Autodesk Fusion 360 part; units mm, degrees
(part 4 of 4)
  constraint vertical L97
  constraint horizontal L47
  constraint vertical L93
  constraint coincident L93.end L232
  constraint coincident L93.end L237
  constraint horizontal L222
  constraint vertical L60
  constraint horizontal L64
  constraint vertical L236
  constraint coincident L222.start L207
  constraint coincident L222.start L231
  constraint horizontal L71
  constraint vertical L234
  constraint horizontal L88
  constraint vertical L148
  constraint coincident L71.start L207
  constraint coincident L71.start L213
  constraint horizontal L81
  constraint vertical L221
  constraint horizontal L149
  constraint vertical L77
  constraint horizontal L65
  constraint vertical L68
  constraint horizontal L66
  constraint vertical L59
  constraint horizontal L104
  constraint vertical L118
  constraint horizontal L18
  constraint vertical L109
  constraint coincident L104.start L207
  constraint coincident L104.start L107
  constraint horizontal L113
  constraint vertical L55
  constraint horizontal L111
  constraint vertical L116
  constraint horizontal L58
  constraint vertical L105
  constraint horizontal L115
  constraint vertical L19
  constraint horizontal L37
  constraint vertical L45
  constraint horizontal L227
  constraint vertical L53
  constraint horizontal L99
  constraint vertical L46
  constraint horizontal L41
  constraint vertical L49
  constraint horizontal L75
  constraint vertical L67
  constraint horizontal L244
  constraint vertical L70
  constraint horizontal L73
  constraint vertical L72
  constraint horizontal L220
  constraint vertical L224
  constraint coincident L73.start L219.start
  constraint coincident P0 L239.start
  constraint perpendicular L223 L239
  constraint coincident A35.centre L240
  constraint coincident A35 L240.end
  constraint coincident A35 L241.start
  constraint collinear L240 L241
  constraint coincident A36.centre L241
  constraint coincident A36 L241.end
  constraint coincident A36 L242.start
  constraint collinear L241 L242
  constraint coincident A37.centre L242
  constraint coincident A37 L242.end
  constraint coincident A37 L243.start
  constraint collinear L242 L243
  constraint coincident A38.centre L243
  constraint coincident A38 L243.end
  constraint coincident A38 L246.start
  constraint collinear L243 L246
  constraint coincident A39.centre L246
  constraint coincident A40.centre L246
  constraint coincident A40 L244.end
  constraint coincident A40 L245.start
  constraint collinear L244 L245
  constraint coincident A40 L246.end
  constraint coincident A40 L247.start
  constraint collinear L246 L247
  measures "d102" distance of L51.end L80.start
  measures "d103" distance of L76.start L80.start
  measures "d104" distance of L128.end L76.start
  measures "d105" distance of L76.start L121.end
  measures "d15" distance of L128.end L78.start
  measures "d16" distance of L78.start L78.end
  measures "d108" distance of L165.end L78.start
  measures "d109" distance of L79.start L78.end
  measures "d110" distance of L79.end L79.start
  measures "d111" distance of L79.start L146.start
  measures "d112" distance of L79.end L9.start
  measures "d113" distance of L9.start L5.start
  measures "d114" distance of L9.start L28.end
  measures "d115" distance of L5.start L10.end
  measures "d116" distance of L10.end L2.start
  measures "d117" distance of L3.end L10.end
  measures "d118" distance of L2.end L2.start
  measures "d119" distance of L15.start L2.end
  measures "d120" distance of L2.end L6.start
  measures "d121" distance of L15.start L106.start
  measures "d122" distance of L15.start L70.end
  measures "d32" distance of L24.end L106.start
  measures "d33" distance of L24.start L14.end
  measures "d34" distance of L14.start L14.end
  measures "d35" distance of L14.start L23.start
  measures "d36" distance of L23.start L54.end
  measures "d37" distance of L54.end L11.start
  measures "d38" distance of L11.start L61.start
  measures "d39" distance of L61.start L8.end
  measures "d40" distance of L59.end L8.end
  measures "d41" distance of L40.end L59.end
  measures "d42" distance of L164.start L164.end
  measures "d43" distance of L164.start L120.end
  measures "d44" distance of L82.start L82.end
  measures "d45" distance of L82.start L167.start
  measures "d46" distance of L161.start L84.start
  measures "d47" distance of L161.start L157.end
  measures "d48" distance of L194.end L199.end
  measures "d49" distance of L194.end L153.end
  measures "d50" distance of L132.start L139.start
  measures "d51" distance of L87.end L139.start
  measures "d52" distance of L135.start L63.end
  measures "d53" distance of L63.start L63.end
  measures "d54" distance of L134.start L134.end
  measures "d55" distance of L134.start L182.end
  measures "d56" distance of L143.start L131.start
  measures "d57" distance of L143.start L125.end
  measures "d58" distance of L163.end L163.start
  measures "d59" distance of L163.start L192.start
  measures "d60" distance of L183.end L138.start
  measures "d61" distance of L183.start L183.end
  measures "d62" distance of L173.start L129.start
  measures "d63" distance of L173.start L158.end
  measures "d64" distance of L187.start L141.start
  measures "d65" distance of L187.start L178.end
  measures "d66" distance of L137.end L137.start
  measures "d67" distance of L154.start L137.start
  measures "d68" distance of L181.end L152.end
  measures "d69" distance of L151.end L152.end
  measures "d70" distance of L166.start L62.end
  measures "d71" distance of L62.start L62.end
  measures "d72" distance of L7.start L7.end
  measures "d73" distance of L7.start L13.start
  measures "d74" distance of L4.end L4.start
  measures "d75" distance of L4.start L29.end
  measures "d76" distance of L57.start L17.start
  measures "d77" distance of L100.start L57.start
  measures "d78" distance of L0.start L21.end
  measures "d79" distance of L21.start L21.end
  measures "d80" distance of L33.end L26.end
  measures "d81" distance of L26.end L1.end
  measures "d82" distance of L36.start L36.end
  measures "d83" distance of L36.start L44.start
  measures "d84" distance of L90.end L52.start
  measures "d85" distance of L90.end L35.end
  measures "d86" distance of L56.end L56.start
  measures "d87" distance of L91.end L56.start
  measures "d88" distance of L93.end L95.end
  measures "d89" distance of L47.end L93.end
  measures "d90" distance of L60.start L222.start
  measures "d91" distance of L64.end L222.start
  measures "d92" distance of L71.end L71.start
  measures "d93" distance of L71.start L88.end
  measures "d94" distance of L81.end L61.start
  measures "d95" distance of L77.start L61.start
  measures "d96" distance of L65.end L59.end
  measures "d97" distance of L59.end L59.start
  measures "d98" distance of L104.end L104.start
  measures "d99" distance of L18.end L104.start
  measures "d100" distance of L55.start L54.end
  measures "d101" distance of L111.end L54.end
  measures "d193" distance of L14.start L58.end
  measures "d194" distance of L14.start L19.start
  measures "d195" distance of L37.start L37.end
  measures "d196" distance of L53.start L37.start
  measures "d106" distance of L49.end L46.start
  measures "d107" distance of L49.end L41.end
  measures "d199" distance of L70.end L67.start
  measures "d200" distance of L70.end L70.start
  measures "d201" distance of L72.start L73.start
  measures "d202" distance of L73.start L220.end
  measures "d203" diameter of A20
  measures "d204" diameter of A22
  measures "d205" diameter of A32
  measures "d206" diameter of A4
  measures "d207" diameter of A13
  measures "d208" diameter of A11
  measures "d209" diameter of A34
  measures "d210" diameter of A9
  measures "d211" diameter of A8
  measures "d212" diameter of A5
  measures "d213" diameter of A12
  measures "d123" diameter of A27
  measures "d124" diameter of A29
  measures "d125" diameter of A24
  measures "d126" diameter of A7
  measures "d127" diameter of A10
  measures "d128" diameter of A33
  measures "d129" diameter of A14
  measures "d130" diameter of A25
  measures "d131" diameter of A28
  measures "d132" diameter of A23
  measures "d133" diameter of A30
  measures "d134" diameter of A26
  measures "d135" diameter of A31
  measures "d136" diameter of A21
  measures "d137" diameter of A18
  measures "d138" diameter of A19
  measures "d139" diameter of A1
  measures "d140" diameter of A3
  measures "d141" diameter of A0
  measures "d142" diameter of A2
  measures "d143" diameter of A15
  measures "d144" diameter of A6
  measures "d145" diameter of A16
  measures "d146" diameter of A17
  measures "d149" distance of A30.centre L128
  measures "d150" distance of A30.centre A31.centre
  measures "d151" distance of A23.centre A31.centre
  measures "d152" distance of A24.centre A23.centre
  measures "d153" distance of A20.centre A24.centre
  measures "d154" distance of A20.centre L137
  measures "d155" distance of A30.centre L210
  measures "d156" distance of A26.centre A30.centre
  measures "d157" distance of A26.centre A18.centre
  measures "d158" distance of A1.centre A18.centre
  measures "d159" distance of A1.centre A0.centre
  measures "d160" distance of A15.centre A0.centre
  measures "d161" distance of A16.centre A15.centre
  measures "d251" distance of P0 L239.end
  measures "d252" diameter of A35
  measures "d253" diameter of A36
  measures "d254" diameter of A37
  measures "d255" diameter of A38
  measures "d256" diameter of A39
  measures "d257" diameter of A40

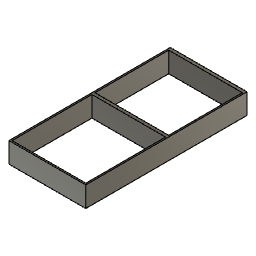
design "Grilla E."
Autodesk Fusion 360 part; units mm, degrees
sketch "Sketch1" plane through (0, 0, 0) normal (0, 0, 1) x (1, 0, 0)
  line L0 (36.035, 36.035) -> (-36.035, 36.035)
  line L1 (-36.035, 36.035) -> (-36.035, -36.035)
  line L2 (-36.035, -36.035) -> (36.035, -36.035)
  line L3 (36.035, -36.035) -> (36.035, 36.035)
  line L4 (36.035, 36.035) -> (-36.035, -36.035) construction
  line L5 (-36.035, 36.035) -> (36.035, -36.035) construction
  line L6 (-36.035, -36.035) -> (36.035, -36.035)
  line L7 (36.035, -39.035) -> (-36.035, -39.035)
  line L8 (-36.035, -39.035) -> (36.035, -39.035)
  line L9 (36.035, -39.035) -> (36.035, -117.035)
  line L10 (36.035, -117.035) -> (-36.035, -117.035)
  line L11 (-36.035, -117.035) -> (-36.035, -39.035)
  line L12 (36.035, 39.035) -> (-36.035, 39.035)
  line L13 (36.035, 39.035) -> (37.465, 39.035)
  line L14 (-37.535, 36.035) -> (-37.535, -36.035)
  line L15 (-37.535, -117.035) -> (-37.535, -39.035)
  line L16 (36.035, -118.535) -> (-36.035, -118.535)
  line L17 (-37.535, 36.035) -> (-37.535, 39.035)
  line L18 (-37.535, 39.035) -> (-36.035, 39.035)
  line L19 (-37.535, -36.035) -> (-37.535, -39.035)
  line L20 (-37.535, -117.035) -> (-37.535, -118.535)
  line L21 (-37.535, -118.535) -> (-36.035, -118.535)
  line L22 (36.035, -118.535) -> (37.465, -118.535)
  line L23 (-37.535, 45.8122) -> (37.465, 45.8122)
  line L24 (37.465, -118.535) -> (37.465, 39.035)
  line L25 (35.965, 36.035) -> (35.965, -36.035)
  dimension "d10" = 72.07
  dimension "d11" = 72.07
  dimension "d12" = 3
  dimension "d13" = 78
  dimension "d16" = 3
  dimension "d17" = 1.5
  dimension "d18" = -1.5
  dimension "d19" = -1.5
  dimension "d23" = 75
  constraint horizontal L0
  constraint perpendicular L0 L1
  constraint parallel L0 L2
  constraint parallel L1 L3
  constraint coincident L4 origin
  constraint coincident L5 origin
  constraint horizontal L6
  constraint horizontal L7
  constraint horizontal L8
  constraint vertical L9
  constraint horizontal L10
  constraint vertical L11
  constraint perpendicular L12 L17
  constraint perpendicular L17 L18
  constraint perpendicular L8 L19
  constraint perpendicular L8 L20
  constraint perpendicular L20 L21
  constraint perpendicular L17 L23
  constraint vertical L24
  constraint coincident L2 L25.end
  constraint coincident L0 L25.start
  measures "d10" distance of L1.end L2.end
  measures "d11" distance of L0.end L1.end
  measures "d12" distance of L1.end L7.end
  measures "d13" distance of L7.end L10.end
  measures "d23" distance of L23.start L23.end
extrude "Extrude2" add sketch "Sketch1" along normal blind 20

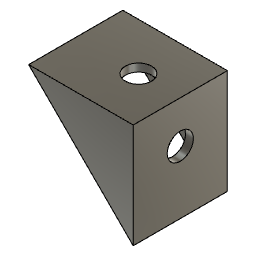
design "F.Escuadra plastica.v3"
Autodesk Fusion 360 part; units mm, degrees
sketch "Sketch1" plane through (0, 0, 0) normal (0, 1, 0) x (1, 0, 0)
  line L0 (10, -10) -> (-10, -10)
  line L1 (10, 10) -> (10, -10)
  line L2 (-10, -10) -> (10, 10) construction
  line L3 (-10, -10) -> (10, 10)
  constraint horizontal L0
  constraint coincident L2 origin
  constraint parallel L2 L3
extrude "Extrude1" add sketch "Sketch1" along normal blind 18
ref_plane "WorkPlane1" through (0, 9, 10) normal (0, 0, 1) x (1, 0, 0)
sketch "Sketch2" plane through (0, 9, 10) normal (0, 0, 1) x (1, 0, 0)
  line L0 (10, 9) -> (-10, -9) construction
  circle A0 centre (2, 0) radius 2.5
  line L1 (10, 9) -> (-10, 9)
  line L2 (10, -9) -> (10, 9)
  line L3 (10, -9) -> (-10, 9) construction
  line L4 (-10, 9) -> (-10, -9)
  line L5 (-10, -9) -> (10, -9)
  point P0 (10, -9)
  dimension "d47" = 20
  dimension "d53" = 5
  dimension "d54" = 18
  dimension "d20" = 8
  dimension "d21" = 9
  constraint perpendicular L1 L2
  constraint parallel L2 L4
  constraint parallel L1 L5
  constraint coincident origin L3
  constraint coincident origin L0
  measures "d47" distance of L1.end L0.start
  measures "d53" diameter of A0
  measures "d54" distance of P0 L0.start
  measures "d20" distance of A0.centre L2
  measures "d21" distance of A0.centre L5
extrude "Extrude2" cut sketch "Sketch2" against normal blind 45 contours A0
ref_plane "WorkPlane2" through (10, 9, 0) normal (1, 0, 0) x (0, 0, -1)
sketch "Sketch3" plane through (10, 9, 0) normal (1, 0, 0) x (0, 1, 0)
  line L0 (-9, 10) -> (9, 10)
  line L1 (0, 10) -> (0, 2)
  circle A0 centre (0, 2) radius 2.5
  dimension "d12" = 8
  dimension "d13" = 5
  dimension "d22" = 9
  constraint midpoint L0 L1.start
  constraint perpendicular L0 L1
  constraint coincident L1.end A0.centre
  measures "d12" distance of L1.start L1.end
  measures "d13" diameter of A0
  measures "d22" horizontal distance of L0.end L1.end
extrude "Extrude3" cut sketch "Sketch3" against normal blind 33
ref_plane "WorkPlane3" through (0, 2, 0) normal (0, -1, 0) x (-1, 0, 0)
sketch "Sketch4" plane through (0, 2, 0) normal (0, -1, 0) x (1, 0, 0)
  line L0 (10, 10) -> (-10, 10)
  line L1 (10, -10) -> (10, 10)
  line L2 (8.5, -6.3787) -> (8.5, 8.5)
  line L3 (8.5, 8.5) -> (-6.3787, 8.5)
  line L4 (-6.3787, 8.5) -> (-10.3794, 8.5)
  line L5 (-10.3794, 8.5) -> (8.5, -10.3794)
  line L6 (8.5, -10.3794) -> (8.5, -6.3787)
  constraint parallel L3 L4
  constraint parallel L2 L6
  constraint parallel L1 L2
  constraint parallel L0 L3
extrude "Extrude4" cut sketch "Sketch4" against normal blind 14

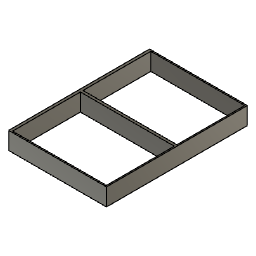
design "Grilla D"
Autodesk Fusion 360 part; units mm, degrees
sketch "Sketch1" plane through (0, 0, 0) normal (0, 0, 1) x (1, 0, 0)
  line L0 (54, 39) -> (-54, 39)
  line L1 (-54, 39) -> (-54, -39)
  line L2 (-54, -39) -> (54, -39)
  line L3 (54, -39) -> (54, 39)
  line L4 (54, 39) -> (-54, -39) construction
  line L5 (-54, 39) -> (54, -39) construction
  line L6 (-54, -39) -> (54, -39)
  line L7 (54, -42) -> (-54, -42)
  line L8 (-54, -42) -> (54, -42)
  line L9 (54, -42) -> (54, -120)
  line L10 (54, -120) -> (-54, -120)
  line L11 (-54, -120) -> (-54, -42)
  line L12 (55.5, -42) -> (55.5, -121.5)
  line L13 (55.5, -121.5) -> (-54, -121.5)
  line L14 (55.5, -39) -> (55.5, 40.5)
  line L15 (55.5, 40.5) -> (-54, 40.5)
  line L16 (55.5, -39) -> (55.5, -42)
  line L17 (-57, 39) -> (-57, -39)
  line L18 (-57, -120) -> (-57, -42)
  line L19 (-57, -120) -> (-57, -121.5)
  line L20 (-57, -121.5) -> (-54, -121.5)
  line L21 (-57, -39) -> (-57, -42)
  line L22 (-54, 40.5) -> (-57, 40.5)
  line L23 (-57, 40.5) -> (-57, 39)
  dimension "d9" = 108
  dimension "d10" = 78
  dimension "d11" = 3
  dimension "d12" = 108
  dimension "d13" = 78
  dimension "d14" = -1.5
  dimension "d15" = 1.5
  dimension "d16" = 3
  dimension "d17" = -3
  constraint horizontal L0
  constraint perpendicular L0 L1
  constraint parallel L0 L2
  constraint parallel L1 L3
  constraint coincident L4 origin
  constraint coincident L5 origin
  constraint horizontal L6
  constraint horizontal L7
  constraint horizontal L8
  constraint vertical L9
  constraint horizontal L10
  constraint vertical L11
  constraint parallel L12 L16
  constraint perpendicular L13 L19
  constraint perpendicular L18 L20
  constraint perpendicular L20 L21
  constraint perpendicular L17 L22
  constraint perpendicular L15 L23
  measures "d9" distance of L1.end L2.end
  measures "d10" distance of L0.end L1.end
  measures "d11" distance of L1.end L7.end
  measures "d12" distance of L7.end L7.start
  measures "d13" distance of L7.end L10.end
extrude "Extrude2" add sketch "Sketch1" along normal blind 20

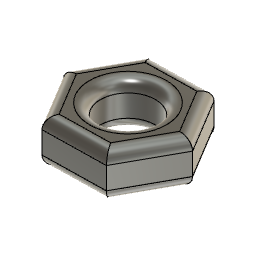
design "N.Perno Alen.v2"
Autodesk Fusion 360 part; units mm, degrees
sketch "Sketch1" plane through (0, 0, 0) normal (0, 0, 1) x (1, 0, 0)
  line L0 (-1.4906, 2.4721) -> (-2.8862, -0.0549)
  line L1 (-2.8862, -0.0549) -> (-1.3956, -2.527)
  line L2 (-1.3956, -2.527) -> (1.4906, -2.4721)
  line L3 (1.4906, -2.4721) -> (2.8862, 0.0549)
  line L4 (2.8862, 0.0549) -> (1.3956, 2.527)
  line L5 (1.3956, 2.527) -> (-1.4906, 2.4721)
  circle A0 centre (0, 0) radius 1.25
  dimension "d1" = 2.5
  dimension "d2" = 2.5
  constraint coincident A0.centre origin
  measures "d1" distance of A0.centre L5
  measures "d2" diameter of A0
extrude "Extrude1" add sketch "Sketch1" along normal blind 2
fillet "Fillet1" radius 0.5 1 faces at (0.0628, -2.0819, 2)
fillet "Fillet2" radius 0.5 1 faces at (0.0628, -2.0819, 0)

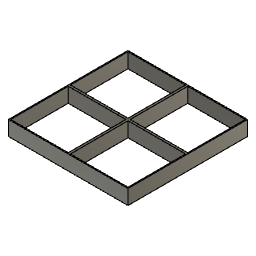
design "Grilla B."
Autodesk Fusion 360 part; units mm, degrees
sketch "Sketch1" plane through (0, 0, 0) normal (0, 0, 1) x (1, 0, 0)
  line L0 (39, 39) -> (-39, 39)
  line L1 (-39, 39) -> (-39, -39)
  line L2 (-39, -39) -> (39, -39)
  line L3 (39, -39) -> (39, 39)
  line L4 (39, 39) -> (-39, -39) construction
  line L5 (-39, 39) -> (39, -39) construction
  line L6 (40.5, -40.5) -> (40.5, 40.5)
  line L7 (40.5, 40.5) -> (-40.5, 40.5)
  line L8 (39, -42) -> (-39, -120) construction
  line L9 (-39, -42) -> (-39, -120)
  line L10 (39, -120) -> (39, -42)
  line L11 (-39, -120) -> (39, -120)
  line L12 (40.5, -121.5) -> (40.5, -40.5)
  line L13 (-39, -42) -> (39, -120) construction
  line L14 (39, -42) -> (-39, -42)
  line L15 (-40.5, -121.5) -> (40.5, -121.5)
  line L16 (-120, -39) -> (-42, -39)
  line L17 (-42, -42) -> (-120, -42)
  line L18 (-121.5, -121.5) -> (-40.5, -121.5)
  line L19 (-121.5, 40.5) -> (-121.5, -40.5)
  line L20 (-120, -120) -> (-42, -120)
  line L21 (-120, -42) -> (-42, -120) construction
  line L22 (-42, -42) -> (-120, -120) construction
  line L23 (-121.5, -40.5) -> (-121.5, -121.5)
  line L24 (-120, 39) -> (-120, -39)
  line L25 (-42, 39) -> (-120, 39)
  line L26 (-120, -42) -> (-120, -120)
  line L27 (-42, -39) -> (-42, 39)
  line L28 (-42, -120) -> (-42, -42)
  line L29 (-120, 39) -> (-42, -39) construction
  line L30 (-42, 39) -> (-120, -39) construction
  line L31 (-40.5, 40.5) -> (-121.5, 40.5)
  point P0 (0, -81)
  point P1 (0, -81)
  point P2 (-81, -81)
  point P3 (-81, 0)
  point P4 (-81, -81)
  point P5 (-81, 0)
  dimension "d1" = 78
  dimension "d2" = 78
  dimension "d4" = 1.5
  dimension "d5" = 78
  dimension "d6" = 78
  dimension "d7" = 1.5
  dimension "d8" = 1.5
  dimension "d9" = 78
  dimension "d10" = 78
  dimension "d11" = 78
  dimension "d12" = 78
  constraint horizontal L0
  constraint perpendicular L0 L1
  constraint parallel L0 L2
  constraint parallel L1 L3
  constraint coincident L4 origin
  constraint coincident L5 origin
  constraint horizontal L14
  constraint perpendicular L9 L14
  constraint parallel L11 L14
  constraint parallel L9 L10
  constraint coincident P1 L8
  constraint coincident P1 L13
  constraint coincident P1 P0
  constraint horizontal L25
  constraint perpendicular L24 L25
  constraint parallel L16 L25
  constraint parallel L24 L27
  constraint coincident P5 L30
  constraint coincident P5 L29
  constraint coincident P5 P3
  constraint horizontal L17
  constraint perpendicular L17 L26
  constraint parallel L17 L20
  constraint parallel L26 L28
  constraint coincident P4 L22
  constraint coincident P4 L21
  constraint coincident P4 P2
  constraint parallel L3 L6
  constraint parallel L0 L7
  constraint parallel L25 L31
  constraint parallel L19 L24
  constraint parallel L18 L20
  constraint parallel L23 L26
  constraint parallel L11 L15
  constraint parallel L10 L12
  measures "d1" distance of L1.end L2.end
  measures "d2" distance of L0.end L1.end
  measures "d5" distance of L10.start L8.end
  measures "d6" distance of L9.start L8.end
  measures "d9" distance of L16.end L16.start
  measures "d10" distance of L24.start L16.start
  measures "d11" distance of L20.start L20.end
  measures "d12" distance of L20.start L17.end
extrude "Extrude1" add sketch "Sketch1" along normal blind 20

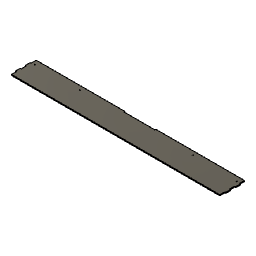
design "B.Borde Seperior e inferior.v3"
Autodesk Fusion 360 part; units mm, degrees
ref_plane "WorkPlane1" through (0, 3, 0) normal (0, 1, 0) x (0, 0, 1)
sketch "Sketch1" plane through (0, 3, 0) normal (0, 1, 0) x (1, 0, 0)
  line L0 (340.5, -241.5) -> (-340.5, -241.5) construction
  line L1 (-340.5, -241.5) -> (-340.5, 241.5) construction
  line L2 (-340.5, 241.5) -> (340.5, 241.5) construction
  line L3 (340.5, 241.5) -> (340.5, -241.5) construction
  line L4 (340.5, -241.5) -> (-340.5, 241.5) construction
  line L5 (-340.5, -241.5) -> (340.5, 241.5) construction
  line L6 (-340.5, -241.5) -> (340.5, -241.5)
  line L7 (340.5, -241.5) -> (340.5, -238.5)
  line L8 (340.5, -238.5) -> (-340.5, -238.5)
  line L9 (-340.5, -238.5) -> (-340.5, -241.5)
  dimension "d2" = 681
  dimension "d3" = 483
  dimension "d4" = 3
  constraint horizontal L0
  constraint perpendicular L0 L1
  constraint parallel L0 L2
  constraint parallel L1 L3
  constraint coincident L4 origin
  constraint coincident L5 origin
  constraint horizontal L6
  constraint vertical L7
  constraint horizontal L8
  constraint vertical L9
  measures "d2" distance of L1.end L2.end
  measures "d3" distance of L0.end L1.end
  measures "d4" distance of L0.end L8.end
  measures "d38" diameter of L7
extrude "Extrude1" add sketch "Sketch1" along normal blind 80
ref_plane "WorkPlane2" through (0, 43, 241.5) normal (0, 0, 1) x (1, 0, 0)
sketch "Sketch2" plane through (0, 42, 241.5) normal (0, 0, 1) x (1, 0, 0)
  line L0 (-340.5, -39) -> (340.5, -39)
  line L1 (340.5, -39) -> (340.5, 41)
  line L2 (340.5, 41) -> (-340.5, 41)
  line L3 (-340.5, 41) -> (-340.5, -39)
  line L4 (-340.5, -39) -> (-337.5, -39)
  line L5 (-337.5, -39) -> (-337.5, -23)
  line L6 (-337.5, -23) -> (-340.5, -23)
  line L7 (-340.5, -23) -> (-340.5, -39)
  line L8 (-340.5, -23) -> (-343.5, -23)
  line L9 (-343.5, -23) -> (-343.5, -7)
  line L10 (-343.5, -7) -> (-340.5, -7)
  line L11 (-340.5, -7) -> (-340.5, -23)
  line L12 (-340.5, -7) -> (-337.5, -7)
  line L13 (-337.5, -7) -> (-337.5, 9)
  line L14 (-337.5, 9) -> (-340.5, 9)
  line L15 (-340.5, 9) -> (-340.5, -7)
  line L16 (-340.5, 9) -> (-343.5, 9)
  line L17 (-343.5, 9) -> (-343.5, 25)
  line L18 (-343.5, 25) -> (-340.5, 25)
  line L19 (-340.5, 25) -> (-340.5, 9)
  line L20 (-340.5, 40) -> (-340.5, 25)
  line L21 (0, 0) -> (0, 41) construction
  line L22 (340.5, -39) -> (337.5, -39)
  line L23 (337.5, -39) -> (337.5, -23)
  line L24 (337.5, -23) -> (340.5, -23)
  line L25 (340.5, -23) -> (340.5, -39)
  line L26 (340.5, -23) -> (343.5, -23)
  line L27 (343.5, -23) -> (343.5, -7)
  line L28 (343.5, -7) -> (340.5, -7)
  line L29 (340.5, -7) -> (340.5, -23)
  line L30 (340.5, -7) -> (337.5, -7)
  line L31 (337.5, -7) -> (337.5, 9)
  line L32 (337.5, 9) -> (340.5, 9)
  line L33 (340.5, 9) -> (340.5, -7)
  line L34 (340.5, 9) -> (343.5, 9)
  line L35 (343.5, 9) -> (343.5, 25)
  line L36 (343.5, 25) -> (340.5, 25)
  line L37 (340.5, 25) -> (340.5, 9)
  line L38 (340.5, 40) -> (340.5, 25)
  line L39 (0, 0) -> (50, 0) construction
  line L40 (0, 0) -> (-50, 0) construction
  line L41 (-50, 41) -> (50, 41)
  line L42 (50, 41) -> (50, 38)
  line L43 (50, 38) -> (-50, 38)
  line L44 (-50, 38) -> (-50, 41)
  line L45 (340.5, 25) -> (337.5, 25)
  line L46 (337.5, 25) -> (337.5, 41)
  line L47 (337.5, 41) -> (340.5, 41)
  line L48 (340.5, 41) -> (340.5, 25)
  line L49 (-340.5, 25) -> (-337.5, 25)
  line L50 (-337.5, 25) -> (-337.5, 41)
  line L51 (-337.5, 41) -> (-340.5, 41)
  line L52 (-340.5, 41) -> (-340.5, 25)
  dimension "d8" = 3
  dimension "d9" = 16
  dimension "d10" = 3
  dimension "d11" = 16
  dimension "d12" = 3
  dimension "d13" = 16
  dimension "d14" = 3
  dimension "d15" = 16
  dimension "d17" = 3
  dimension "d18" = 16
  dimension "d19" = 3
  dimension "d20" = 16
  dimension "d21" = 3
  dimension "d22" = 16
  dimension "d23" = 3
  dimension "d24" = 16
  dimension "d26" = 50
  dimension "d27" = 50
  dimension "d28" = 3
  dimension "d31" = 3
  constraint horizontal L4
  constraint vertical L5
  constraint horizontal L6
  constraint vertical L7
  constraint coincident L0.start L3.end
  constraint horizontal L8
  constraint vertical L9
  constraint horizontal L10
  constraint vertical L11
  constraint horizontal L12
  constraint vertical L13
  constraint horizontal L14
  constraint vertical L15
  constraint horizontal L16
  constraint vertical L17
  constraint horizontal L18
  constraint vertical L19
  constraint vertical L20
  constraint coincident L21.start L39.start
  constraint midpoint L2 L21.end
  constraint horizontal L22
  constraint vertical L23
  constraint horizontal L24
  constraint vertical L25
  constraint coincident L0.end L1.start
  constraint horizontal L26
  constraint vertical L27
  constraint horizontal L28
  constraint vertical L29
  constraint horizontal L30
  constraint vertical L31
  constraint horizontal L32
  constraint vertical L33
  constraint horizontal L34
  constraint vertical L35
  constraint horizontal L36
  constraint vertical L37
  constraint vertical L38
  constraint perpendicular L21 L39
  constraint perpendicular L21 L40
  constraint horizontal L41
  constraint vertical L42
  constraint horizontal L43
  constraint vertical L44
  constraint coincident L2 L41.start
  constraint horizontal L45
  constraint vertical L46
  constraint horizontal L47
  constraint vertical L48
  constraint coincident L2 L46.end
  constraint horizontal L49
  constraint vertical L50
  constraint horizontal L51
  constraint vertical L52
  measures "d8" distance of L0.start L4.end
  measures "d9" distance of L0.start L6.end
  measures "d10" distance of L6.end L8.end
  measures "d11" distance of L6.end L10.end
  measures "d12" distance of L10.end L12.end
  measures "d13" distance of L10.end L14.end
  measures "d14" distance of L14.end L16.end
  measures "d15" distance of L14.end L18.end
  measures "d17" distance of L0.end L22.end
  measures "d18" distance of L0.end L24.end
  measures "d19" distance of L24.end L26.end
  measures "d20" distance of L24.end L28.end
  measures "d21" distance of L28.end L30.end
  measures "d22" distance of L28.end L32.end
  measures "d23" distance of L32.end L34.end
  measures "d24" distance of L32.end L36.end
  measures "d26" distance of L21.start L39.end
  measures "d27" distance of L21.start L40.end
  measures "d28" distance of L41.start L43.end
  measures "d31" distance of L18.end L49.end
extrude "Extrude2" cut sketch "Sketch2" against normal blind 50 contours L0 L3 L4 L5 L6 L7 | L0 L1 L22 L23 L24 L25 | L3 L12 L13 L14 L15 | L2 L3 L20 L49 L50 L51 L52 | L1 L30 L31 L32 L33 | L1 L2 L38 L45 L46 L47 L48 | L2 L41 L42 L43 L44
ref_plane "WorkPlane3" through (0, 43, 241.5) normal (0, 0, 1) x (1, 0, 0)
sketch "Sketch3" plane through (0, 43, 241.5) normal (0, 0, 1) x (1, 0, 0)
  line L0 (337.5, 8) -> (340.5, 8)
  line L1 (340.5, 8) -> (340.5, 24)
  line L2 (340.5, 24) -> (337.5, 24)
  line L3 (337.5, 24) -> (337.5, 40)
  line L4 (337.5, 40) -> (50, 40)
  line L5 (50, 40) -> (50, 37)
  line L6 (50, 37) -> (-50, 37)
  line L7 (-50, 37) -> (-50, 40)
  line L8 (-50, 40) -> (-337.5, 40)
  line L9 (-337.5, 40) -> (-337.5, 24)
  line L10 (-337.5, 24) -> (-340.5, 24)
  line L11 (-340.5, 24) -> (-340.5, 8)
  line L12 (-340.5, 8) -> (-337.5, 8)
  line L13 (-337.5, 8) -> (-337.5, -8)
  line L14 (-337.5, -8) -> (-340.5, -8)
  line L15 (-340.5, -8) -> (-340.5, -24)
  line L16 (-340.5, -24) -> (-337.5, -24)
  line L17 (-337.5, -24) -> (-337.5, -40)
  line L18 (-337.5, -40) -> (337.5, -40)
  line L19 (337.5, -40) -> (337.5, -24)
  line L20 (337.5, -24) -> (340.5, -24)
  line L21 (340.5, -24) -> (340.5, -8)
  line L22 (340.5, -8) -> (337.5, -8)
  line L23 (337.5, -8) -> (337.5, 8)
ref_plane "WorkPlane4" through (0, 43, 241.5) normal (0, 0, 1) x (1, 0, 0)
sketch "Sketch4" plane through (0, 43, 241.5) normal (0, 0, 1) x (1, 0, 0)
  circle A0 centre (327.5, 25) radius 1.5
  line L0 (-337.5, -40) -> (-317.5, -40) construction
  line L1 (-50, 37) -> (-224.7348, 37)
  line L2 (50, 37) -> (230, 37) construction
  line L3 (177.5, 19) -> (197.5, 19)
  line L4 (177.5, 37) -> (177.5, 19)
  line L5 (197.5, 19) -> (197.5, 37)
  circle A1 centre (183.022, 27) radius 1.5
  line L6 (177.5, 19) -> (197.5, 37) construction
  line L7 (197.5, 37) -> (177.5, 37)
  line L8 (177.5, 37) -> (197.5, 19) construction
  line L9 (-337.5, 44.2221) -> (-197.5, 44.2221)
  line L10 (-197.5, 44.2221) -> (-197.5, 37)
  line L11 (0, 0) -> (0, 16.7739)
  line L12 (177.5, 37) -> (197.5, 19) construction
  line L13 (177.5, 19) -> (197.5, 37) construction
  line L14 (197.5, 19) -> (197.5, 37)
  line L15 (197.5, 37) -> (177.5, 37)
  line L16 (177.5, 37) -> (177.5, 19)
  line L17 (177.5, 19) -> (197.5, 19)
  line L18 (-177.5, 37) -> (-177.5, 19)
  circle A2 centre (-183.022, 27) radius 1.5
  line L19 (-197.5, 19) -> (-197.5, 37)
  line L20 (-197.5, 19) -> (-197.5, 37)
  line L21 (-197.5, 37) -> (-177.5, 37)
  line L22 (-177.5, 19) -> (-197.5, 19)
  line L23 (-177.5, 19) -> (-197.5, 37) construction
  line L24 (-177.5, 37) -> (-177.5, 19)
  line L25 (-177.5, 37) -> (-197.5, 19) construction
  line L26 (-197.5, 37) -> (-177.5, 37)
  line L27 (-177.5, 19) -> (-197.5, 37) construction
  line L28 (-177.5, 19) -> (-197.5, 19)
  line L29 (-177.5, 37) -> (-197.5, 19) construction
  line L30 (337.5, 24) -> (337.5, 40)
  line L31 (337.5, 19) -> (317.5, 19)
  line L32 (317.5, 19) -> (317.5, 37)
  line L33 (317.5, 37) -> (337.5, 37)
  line L34 (337.5, 37) -> (337.5, 19)
  line L35 (230, 37) -> (360, 37) construction
  circle A3 centre (-327.5, 25) radius 1.5
  line L36 (-317.5, 19) -> (-317.5, 37)
  line L37 (-337.5, 37) -> (-337.5, 19)
  line L38 (-317.5, 37) -> (-337.5, 37)
  line L39 (-337.5, 19) -> (-317.5, 19)
  line L40 (340.5, 8) -> (340.5, 24)
  line L41 (340.5, 28.005) -> (327.5, 28.005)
  line L42 (50, 40) -> (337.5, 40)
  line L43 (327.5, 40) -> (327.5, 25)
  line L44 (337.5, 40) -> (349, 40)
  line L45 (340.5, 24) -> (340.5, 42)
  line L46 (340.5, 40) -> (327.5, 40)
  line L47 (327.5, 40) -> (327.5, 25)
  line L48 (327.5, 25) -> (340.5, 25)
  line L49 (340.5, 25) -> (340.5, 40)
  line L50 (-340.5, 8) -> (-340.5, 24)
  line L51 (-337.5, 40) -> (-50, 40)
  line L52 (-340.5, 24) -> (-340.5, 44.2221)
  line L53 (-337.5, 40) -> (-349, 40)
  line L54 (-340.5, 40) -> (-327.5, 40)
  line L55 (-327.5, 40) -> (-327.5, 25)
  line L56 (-327.5, 25) -> (-340.5, 25)
  line L57 (-340.5, 25) -> (-340.5, 40)
  line L58 (-185.5, 40) -> (-185.5, 27)
  line L59 (185.5, 40) -> (185.5, 27)
  line L60 (340.5, 24) -> (183.022, 24)
  line L61 (-340.5, 8) -> (-183.022, 8)
  line L62 (-340.5, 49.3423) -> (-183.022, 49.3423)
  point P0 (-327.5, -3)
  point P1 (327.5, -3)
  point P2 (-50, 37)
  point P3 (50, 37)
  point P4 (187.5, 28)
  point P5 (187.5, 28)
  point P6 (197.5, 37)
  point P7 (-187.5, 28)
  point P8 (-197.5, 37)
  point P9 (-187.5, 28)
  point P10 (-197.5, 37)
  point P11 (337.5, 37)
  point P12 (-337.5, 24)
  point P13 (-337.5, 37)
  point P14 (183.022, 27)
  point P15 (-183.022, 27)
  dimension "d38" = 3
  dimension "d47" = 20
  dimension "d53" = 3
  dimension "d55" = 140
  dimension "d56" = 20
  dimension "d60" = 3
  dimension "d63" = 18
  dimension "d64" = 13
  dimension "d65" = 15
  dimension "d66" = 13
  dimension "d67" = 15
  dimension "d68" = 13
  dimension "d69" = 13
  dimension "d70" = 13
  dimension "d71" = 15
  dimension "d73" = 157.478
  dimension "d74" = 157.478
  dimension "d75" = 157.478
  dimension "d76" = 157.478
  constraint coincident P2 L1.start
  constraint horizontal L1
  constraint coincident P3 L2.start
  constraint parallel L1 L2
  constraint perpendicular L3 L4
  constraint parallel L4 L5
  constraint parallel L3 L7
  constraint coincident P5 L8
  constraint coincident P5 L6
  constraint horizontal L9
  constraint coincident L1 P10
  constraint perpendicular L1 L10
  constraint coincident L11.start origin
  constraint vertical L11
  constraint perpendicular L16 L17
  constraint parallel L14 L16
  constraint parallel L15 L17
  constraint coincident P5 L12
  constraint coincident P5 L13
  constraint symmetric L3.end L11 L19.start
  constraint symmetric L4.start L11 L18.start
  constraint symmetric P6 L11 P10
  constraint symmetric P5 L11 P9
  constraint symmetric L3.start L11 L18.end
  constraint symmetric L11 P6 P10
  constraint symmetric L11 L3.end L19.start
  constraint symmetric L11 P5 P9
  constraint symmetric L11 L3.start L18.end
  constraint symmetric L11 L4.start L18.start
  constraint horizontal L31
  constraint vertical L32
  constraint horizontal L33
  constraint vertical L34
  constraint perpendicular L30 L35
  constraint coincident L35 P11
  constraint coincident L30 P11
  constraint symmetric A0 L11 A3
  constraint symmetric L11 L30.start P12
  constraint symmetric L11 L31.start L37.end
  constraint symmetric L11 L31.end L36.start
  constraint symmetric L11 L32.end L36.end
  constraint symmetric L11 P11 P13
  constraint perpendicular L34 L41
  constraint coincident L42 L43.start
  constraint perpendicular L42 L43
  constraint coincident L30.end L42.end
  constraint perpendicular L30 L44
  constraint coincident L40.end L45.start
  constraint perpendicular L44 L45
  constraint horizontal L46
  constraint vertical L47
  constraint horizontal L48
  constraint vertical L49
  constraint coincident A0.centre L43.end
  constraint coincident L45 L46.start
  constraint coincident L44 L46.start
  constraint coincident L50.end L52.start
  constraint perpendicular L38 L52
  constraint coincident L51.start L53.start
  constraint perpendicular L52 L53
  constraint horizontal L54
  constraint vertical L55
  constraint horizontal L56
  constraint vertical L57
  constraint coincident L53 L54.start
  constraint coincident L52 L54.start
  constraint coincident L51 L58.start
  constraint perpendicular L51 L58
  constraint coincident L42 L59.start
  constraint perpendicular L42 L59
  constraint perpendicular L49 L60
  constraint coincident L50.start L61.start
  constraint perpendicular L50 L61
  constraint perpendicular L52 L62
  measures "d38" diameter of A0
  measures "d47" distance of L3.end L3.start
  measures "d53" diameter of A1
  measures "d55" distance of L9.start L9.end
  measures "d56" distance of L3.end L3.start
  measures "d60" diameter of A2
  measures "d63" distance of L31.start P11
  measures "d64" distance of L41.start L41.end
  measures "d65" distance of L43.start A0.centre
  measures "d66" distance of L54.start L54.end
  measures "d67" distance of L54.start L56.end
  measures "d68" distance of L58.start L58.end
  measures "d69" distance of L59.start L59.end
  measures "d70" distance of L40 A0.centre
  measures "d71" distance of A0.centre L46
  measures "d73" distance of L40.end L60.end
  measures "d74" distance of L50.start L61.end
  measures "d75" distance of L62.start L62.end
  measures "d76" horizontal distance of L46.start P14
extrude "Extrude3" cut sketch "Sketch4" against normal blind 100 contours A0 L43 L47 L48 | A0 L43 L47 L48 L60 | A0 L60 | A1 | A2 | A3 L55 L56 | A3 L55 L56

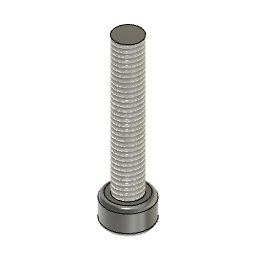
design "M.Perno alen.v2"
Autodesk Fusion 360 part; units mm, degrees
sketch "Sketch1" plane through (0, 0, 0) normal (0, 0, 1) x (1, 0, 0)
  circle A0 centre (0, 0) radius 2.5
  dimension "d1" = 5
  constraint coincident A0.centre origin
  measures "d1" diameter of A0
extrude "Extrude1" add sketch "Sketch1" along normal blind 3
ref_plane "WorkPlane1" through (0, 0, 3) normal (0, 0, 1) x (1, 0, 0)
sketch "Sketch2" plane through (0, 0, 3) normal (0, 0, 1) x (1, 0, 0)
  circle A0 centre (0, 0) radius 1.5
  dimension "d5" = 3
  constraint coincident A0.centre origin
  measures "d5" diameter of A0
extrude "Extrude2" add sketch "Sketch2" along normal blind 16
fillet "Fillet1" radius 0.5 1 edges at (-2.3308, -0.904, 0)
fillet "Fillet2" radius 0.5 1 edges at (-2.3308, -0.904, 3)
thread "Thread1" "ISO Metric profile 3.0 M3x0.5 6g" major diameter 2.927 minor diameter 2.3555 pitch 0.5 angle 60 resizes the face on face at (1.4981, -0.0748, 13.6667)
ref_plane "WorkPlane2" through (0, 0, 0) normal (0, 0, -1) x (-1, 0, 0)
sketch "Sketch3" plane through (0, 0, 0) normal (0, 0, -1) x (1, 0, 0)
  line L0 (-0.866, 1.5) -> (-1.7321, 0)
  line L1 (-1.7321, 0) -> (-0.866, -1.5)
  line L2 (-0.866, -1.5) -> (0.866, -1.5)
  line L3 (0.866, -1.5) -> (1.7321, 0)
  line L4 (1.7321, 0) -> (0.866, 1.5)
  line L5 (0.866, 1.5) -> (-0.866, 1.5)
  dimension "d13" = 1.5
  measures "d13" distance of origin L5
extrude "Extrude3" cut sketch "Sketch3" against normal blind 1

design "C.Bordes Laterales.v3"
Autodesk Fusion 360 part; units mm, degrees
ref_plane "WorkPlane1" through (0, 3, 0) normal (0, 1, 0) x (0, 0, 1)
sketch "Sketch1" plane through (0, 3, 0) normal (0, 1, 0) x (1, 0, 0)
  line L0 (340.5, 241.5) -> (-340.5, 241.5) construction
  line L1 (-340.5, 241.5) -> (-340.5, -241.5) construction
  line L2 (-340.5, -241.5) -> (340.5, -241.5) construction
  line L3 (340.5, -241.5) -> (340.5, 241.5) construction
  line L4 (340.5, 241.5) -> (-340.5, -241.5) construction
  line L5 (-340.5, 241.5) -> (340.5, -241.5) construction
  line L6 (-340.5, 241.5) -> (-337.5, 241.5)
  line L7 (-337.5, 241.5) -> (-337.5, -241.5)
  line L8 (-337.5, -241.5) -> (-340.5, -241.5)
  line L9 (-340.5, -241.5) -> (-340.5, 241.5)
  dimension "d2" = 681
  dimension "d3" = 483
  dimension "d4" = 3
  constraint horizontal L0
  constraint perpendicular L0 L1
  constraint parallel L0 L2
  constraint parallel L1 L3
  constraint coincident L4 origin
  constraint coincident L5 origin
  constraint horizontal L6
  constraint vertical L7
  constraint horizontal L8
  constraint vertical L9
  measures "d2" distance of L1.end L2.end
  measures "d3" distance of L0.end L1.end
  measures "d4" distance of L0.end L6.end
extrude "Extrude1" add sketch "Sketch1" along normal blind 80
ref_plane "WorkPlane2" through (-340.5, 43, 0) normal (-1, 0, 0) x (0, 0, 1)
sketch "Sketch2" plane through (-340.5, 42, 0) normal (-1, 0, 0) x (0, 1, 0)
  line L0 (-39, 241.5) -> (-39, -241.5)
  line L1 (-39, -241.5) -> (41, -241.5)
  line L2 (41, -241.5) -> (41, 241.5)
  line L3 (41, 241.5) -> (-39, 241.5)
  line L4 (0, 0) -> (0, -50) construction
  line L5 (0, 0) -> (0, 50) construction
  line L6 (41, 50) -> (38, 50)
  line L7 (38, 50) -> (38, -50)
  line L8 (38, -50) -> (41, -50)
  line L9 (41, -50) -> (41, 50)
  line L10 (-39, 241.5) -> (-23, 241.5)
  line L11 (-23, 241.5) -> (-23, 244.5)
  line L12 (-23, 244.5) -> (-39, 244.5)
  line L13 (-39, 244.5) -> (-39, 241.5)
  line L14 (-23, 241.5) -> (-7, 241.5)
  line L15 (-7, 241.5) -> (-7, 238.5)
  line L16 (-7, 238.5) -> (-23, 238.5)
  line L17 (-23, 238.5) -> (-23, 241.5)
  line L18 (-7, 241.5) -> (9, 241.5)
  line L19 (9, 241.5) -> (9, 244.5)
  line L20 (9, 244.5) -> (-7, 244.5)
  line L21 (-7, 244.5) -> (-7, 241.5)
  line L22 (9, 241.5) -> (25, 241.5)
  line L23 (25, 241.5) -> (25, 238.5)
  line L24 (25, 238.5) -> (9, 238.5)
  line L25 (9, 238.5) -> (9, 241.5)
  line L26 (-39, -241.5) -> (-23, -241.5)
  line L27 (-23, -241.5) -> (-23, -244.5)
  line L28 (-23, -244.5) -> (-39, -244.5)
  line L29 (-39, -244.5) -> (-39, -241.5)
  line L30 (-23, -241.5) -> (-7, -241.5)
  line L31 (-7, -241.5) -> (-7, -238.5)
  line L32 (-7, -238.5) -> (-23, -238.5)
  line L33 (-23, -238.5) -> (-23, -241.5)
  line L34 (-7, -241.5) -> (9, -241.5)
  line L35 (9, -241.5) -> (9, -244.5)
  line L36 (9, -244.5) -> (-7, -244.5)
  line L37 (-7, -244.5) -> (-7, -241.5)
  line L38 (9, -241.5) -> (25, -241.5)
  line L39 (25, -241.5) -> (25, -238.5)
  line L40 (25, -238.5) -> (9, -238.5)
  line L41 (9, -238.5) -> (9, -241.5)
  line L42 (25, -241.5) -> (40, -241.5)
  line L43 (25, -241.5) -> (41, -241.5)
  line L44 (41, -241.5) -> (41, -244.5)
  line L45 (41, -244.5) -> (25, -244.5)
  line L46 (25, -244.5) -> (25, -241.5)
  line L47 (25, 241.5) -> (41, 241.5)
  line L48 (41, 241.5) -> (41, 244.5)
  line L49 (41, 244.5) -> (25, 244.5)
  line L50 (25, 244.5) -> (25, 241.5)
  dimension "d8" = 50
  dimension "d9" = 50
  dimension "d10" = 3
  dimension "d11" = 16
  dimension "d12" = 3
  dimension "d13" = 16
  dimension "d14" = 3
  dimension "d15" = 16
  dimension "d16" = 3
  dimension "d17" = 16
  dimension "d18" = 3
  dimension "d20" = 16
  dimension "d21" = 3
  dimension "d22" = 16
  dimension "d23" = 3
  dimension "d24" = 16
  dimension "d25" = 3
  dimension "d26" = 16
  dimension "d27" = 3
  dimension "d31" = 3
  dimension "d32" = 3
  constraint coincident L4.start L5.start
  constraint parallel L0 L4
  constraint vertical L5
  constraint horizontal L6
  constraint vertical L7
  constraint horizontal L8
  constraint vertical L9
  constraint coincident L2 L6.start
  constraint horizontal L10
  constraint vertical L11
  constraint horizontal L12
  constraint vertical L13
  constraint coincident L0.start L3.end
  constraint horizontal L14
  constraint vertical L15
  constraint horizontal L16
  constraint vertical L17
  constraint horizontal L18
  constraint vertical L19
  constraint horizontal L20
  constraint vertical L21
  constraint horizontal L22
  constraint vertical L23
  constraint horizontal L24
  constraint vertical L25
  constraint horizontal L26
  constraint vertical L27
  constraint horizontal L28
  constraint vertical L29
  constraint coincident L0.end L1.start
  constraint horizontal L30
  constraint vertical L31
  constraint horizontal L32
  constraint vertical L33
  constraint horizontal L34
  constraint vertical L35
  constraint horizontal L36
  constraint vertical L37
  constraint horizontal L38
  constraint vertical L39
  constraint horizontal L40
  constraint vertical L41
  constraint horizontal L42
  constraint horizontal L43
  constraint vertical L44
  constraint horizontal L45
  constraint vertical L46
  constraint horizontal L47
  constraint vertical L48
  constraint horizontal L49
  constraint vertical L50
  measures "d8" distance of L4.start L4.end
  measures "d9" distance of L4.start L5.end
  measures "d10" distance of L6.start L6.end
  measures "d11" distance of L0.start L10.end
  measures "d12" distance of L0.start L12.end
  measures "d13" distance of L10.end L14.end
  measures "d14" distance of L10.end L16.end
  measures "d15" distance of L14.end L18.end
  measures "d16" distance of L14.end L20.end
  measures "d17" distance of L18.end L22.end
  measures "d18" distance of L18.end L24.end
  measures "d20" distance of L0.end L26.end
  measures "d21" distance of L0.end L28.end
  measures "d22" distance of L26.end L30.end
  measures "d23" distance of L26.end L32.end
  measures "d24" distance of L30.end L34.end
  measures "d25" distance of L30.end L36.end
  measures "d26" distance of L34.end L38.end
  measures "d27" distance of L34.end L40.end
  measures "d31" distance of L38.end L45.end
  measures "d32" distance of L22.end L49.end
extrude "Extrude2" cut sketch "Sketch2" against normal blind 25 contours L3 L14 L15 L16 L17 | L1 L30 L31 L32 L33 | L3 L22 L23 L24 L25 | L1 L38 L39 L40 L41 | L2 L6 L7 L8 L9
ref_plane "WorkPlane3" through (-337.5, 43, 0) normal (1, 0, 0) x (0, 0, -1)
sketch "Sketch3" plane through (-337.5, 43, 0) normal (1, 0, 0) x (0, 1, 0)
  line L0 (37, 50) -> (40, 50)
  line L1 (40, 50) -> (40, 241.5)
  line L2 (40, 241.5) -> (24, 241.5)
  line L3 (24, 241.5) -> (24, 238.5)
  line L4 (24, 238.5) -> (8, 238.5)
  line L5 (8, 238.5) -> (8, 241.5)
  line L6 (8, 241.5) -> (-8, 241.5)
  line L7 (-8, 241.5) -> (-8, 238.5)
  line L8 (-8, 238.5) -> (-24, 238.5)
  line L9 (-24, 238.5) -> (-24, 241.5)
  line L10 (-24, 241.5) -> (-40, 241.5)
  line L11 (-40, 241.5) -> (-40, -241.5)
  line L12 (-40, -241.5) -> (-24, -241.5)
  line L13 (-24, -241.5) -> (-24, -238.5)
  line L14 (-24, -238.5) -> (-8, -238.5)
  line L15 (-8, -238.5) -> (-8, -241.5)
  line L16 (-8, -241.5) -> (8, -241.5)
  line L17 (8, -241.5) -> (8, -238.5)
  line L18 (8, -238.5) -> (24, -238.5)
  line L19 (24, -238.5) -> (24, -241.5)
  line L20 (24, -241.5) -> (40, -241.5)
  line L21 (40, -241.5) -> (40, -50)
  line L22 (40, -50) -> (37, -50)
  line L23 (37, -50) -> (37, 50)
ref_plane "WorkPlane4" through (-337.5, 43, 0) normal (1, 0, 0) x (0, 0, -1)
sketch "Sketch4" plane through (-337.5, 43, 0) normal (1, 0, 0) x (0, 1, 0)
  line L0 (19, 218.5) -> (37, 218.5)
  line L1 (19, -238.5) -> (19, -218.5)
  line L2 (19, -10) -> (37, -10)
  line L3 (45, 241.5) -> (45, 141.5)
  line L4 (24, 241.5) -> (40, 241.5)
  line L5 (37, 141.5) -> (37, 161.5)
  line L6 (28, 241.5) -> (28, 228.5)
  line L7 (40, 241.5) -> (40, 50)
  line L8 (40, -50) -> (40, -241.5)
  line L9 (19, 10) -> (19, -10)
  line L10 (37, -218.5) -> (37, -238.5)
  line L11 (37, 10) -> (19, -10) construction
  line L12 (40, 241.5) -> (45, 241.5)
  line L13 (19, -218.5) -> (37, -218.5)
  line L14 (37, 10) -> (19, 10)
  line L15 (19, 10) -> (37, -10) construction
  line L16 (37, 161.5) -> (19, 161.5)
  circle A0 centre (24, -228.5) radius 1.5
  line L17 (37, 50) -> (37, 260) construction
  line L18 (19, 238.5) -> (19, 218.5)
  circle A1 centre (25, 2) radius 1.5
  line L19 (19, 141.5) -> (37, 141.5)
  line L20 (37, 238.5) -> (19, 238.5)
  line L21 (0, 0) -> (6.2879, 0)
  line L22 (24, -241.5) -> (40, -241.5)
  line L23 (37, -50) -> (37, 50)
  line L24 (42, 238.5) -> (42, 161.5)
  circle A2 centre (24, 228.5) radius 1.5
  line L25 (37, -238.5) -> (19, -238.5)
  line L26 (37, -10) -> (37, 10)
  circle A3 centre (26, 159.346) radius 1.5
  line L27 (37, 238.5) -> (42, 238.5)
  line L28 (19, 161.5) -> (19, 141.5)
  line L29 (37, 218.5) -> (37, 238.5)
  line L30 (37, 50) -> (40, 50)
  line L31 (40, 50) -> (40, 241.5)
  line L32 (40, 241.5) -> (24, 241.5)
  line L33 (24, 241.5) -> (24, 238.5)
  line L34 (24, 238.5) -> (8, 238.5)
  line L35 (8, 238.5) -> (8, 241.5)
  line L36 (8, 241.5) -> (-8, 241.5)
  line L37 (-8, 241.5) -> (-8, 238.5)
  line L38 (-8, 238.5) -> (-24, 238.5)
  line L39 (-24, 238.5) -> (-24, 241.5)
  line L40 (-24, 241.5) -> (-40, 241.5)
  line L41 (-40, 241.5) -> (-40, -241.5)
  line L42 (-40, -241.5) -> (-24, -241.5)
  line L43 (-24, -241.5) -> (-24, -238.5)
  line L44 (-24, -238.5) -> (-8, -238.5)
  line L45 (-8, -238.5) -> (-8, -241.5)
  line L46 (-8, -241.5) -> (8, -241.5)
  line L47 (8, -241.5) -> (8, -238.5)
  line L48 (8, -238.5) -> (24, -238.5)
  line L49 (24, -238.5) -> (24, -241.5)
  line L50 (24, -241.5) -> (40, -241.5)
  line L51 (40, -241.5) -> (40, -50)
  line L52 (40, -50) -> (37, -50)
  line L53 (37, -50) -> (37, 50)
  line L54 (85.1085, 241.5) -> (85.1085, 159.346)
  line L55 (85.1085, 159.346) -> (-10, 159.346)
  point P0 (-0.5, -125.5)
  point P1 (40, 241.5)
  point P2 (37, 238.5)
  point P3 (37, -238.5)
  point P4 (28, 0)
  point P5 (26, 159.346)
  dimension "d47" = 20
  dimension "d53" = 3
  dimension "d54" = 18
  dimension "d64" = 3
  dimension "d65" = 18
  dimension "d66" = 100
  dimension "d67" = 3
  dimension "d68" = 18
  dimension "d69" = 77
  dimension "d70" = 13
  dimension "d71" = 16
  dimension "d72" = 13
  dimension "d73" = 12
  dimension "d74" = 14
  dimension "d75" = 12
  dimension "d93" = 82.154
  constraint horizontal L14
  constraint perpendicular L9 L14
  constraint parallel L2 L14
  constraint parallel L9 L26
  constraint coincident P4 L11
  constraint coincident P4 L15
  constraint horizontal L20
  constraint vertical L18
  constraint horizontal L0
  constraint vertical L29
  constraint coincident L21.start origin
  constraint horizontal L21
  constraint symmetric P2 P3 L21
  constraint symmetric L1.end L0.start L21
  constraint symmetric L18.start L1.start L21
  constraint symmetric L10.start L0.end L21
  constraint symmetric A0 L21 A2
  constraint coincident P1 L4.end
  constraint perpendicular L12 L17
  constraint perpendicular L3 L20
  constraint horizontal L16
  constraint vertical L28
  constraint horizontal L19
  constraint vertical L5
  constraint coincident P2 L20.start
  constraint perpendicular L27 L29
  constraint perpendicular L16 L24
  constraint coincident L6.start L4
  constraint perpendicular L4 L6
  constraint perpendicular L12 L54
  constraint perpendicular L54 L55
  constraint coincident L55 P5
  measures "d47" distance of L2.start L9.start
  measures "d53" diameter of A1
  measures "d54" distance of L11.start L9.start
  measures "d64" diameter of A2
  measures "d65" distance of P2 L18.start
  measures "d66" distance of L3.end L3.start
  measures "d67" diameter of A3
  measures "d68" distance of L16.end L5.end
  measures "d69" distance of L24.end L24.start
  measures "d70" distance of L6.start L6.end
  measures "d71" distance of A0.centre L8
  measures "d72" distance of A0.centre L22
  measures "d73" distance of A1.centre L26
  measures "d74" distance of P5 L7
  measures "d75" distance of L6.end L7
  measures "d93" distance of L54.start L54.end
extrude "Extrude4" cut sketch "Sketch4" against normal blind 45 contours A3 L55 | A3 L55 | A0 | A1 | A2
